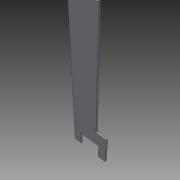
# Autodesk Inventor part: inner_brace_left
Saved by Autodesk Inventor 2014 (Build 180170000, 170)
## iProperties
Created: 2014-03-31
Part Number: inner_brace_left
Material: Generic
Document SubType Name: Modeling
Designer: buben
Density: 1 g/cm^3
Appearance: Default
Author: buben
Autodesk Inventor part; units mm, degrees
ref_plane "YZ Plane" through (0, 0, 0) normal (1, 0, 0) x (0, 1, 0)
ref_plane "XZ Plane" through (0, 0, 0) normal (0, 1, 0) x (-1, 0, 0)
ref_plane "XY Plane" through (0, 0, 0) normal (0, 0, 1) x (1, 0, 0)
sketch "Sketch1" plane through (0, 0, 0) normal (0, 1, 0) x (-1, 0, 0)
  line L0 (0, 0) -> (-100, 0)
  line L1 (0, -489) -> (0, 0)
  line L2 (-30.25, -489) -> (-30.25, -439)
  line L3 (-30.25, -439) -> (-112.25, -439)
  line L4 (-112.25, -439) -> (-112.25, -489)
  line L5 (-142.5, -489) -> (-112.25, -489)
  line L6 (-30.25, -489) -> (0, -489)
  line L7 (-142.5, -489) -> (-142.5, -389)
  line L8 (-142.5, -389) -> (-100, -389)
  line L9 (-100, -389) -> (-100, 0)
  dimension "d0" = 82
  dimension "d1" = 100
  dimension "d2" = 489
  dimension "d3" = 30.25
  dimension "d4" = 50
  dimension "d5" = 50
  constraints: 20 end point, 5 perpendicular, 4 parallel, 2 collinear, 1 horizontal, 1 vertical
  measures "d0" distance of L2.end L3.end
  measures "d1" distance of L0.start L0.end
  measures "d2" distance of L1.start L0.start
  measures "d3" distance of L2.start L1.start
  measures "d4" distance of L2.start L2.end
  measures "d5" distance between parallel lines of L3 L8
extrude "Extrusion1" add sketch "Sketch1" along normal blind 6.5
body "Solid1"
